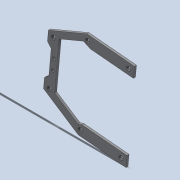
# Autodesk Inventor part: MuzzleHeadMount
Saved by Autodesk Inventor 2020 (Build 240168000, 168)
## iProperties
Created: 2021-07-18
Part Number: MuzzleHeadMount
Material: Generic
Document SubType Name: Sheet Metal
Designer: valer
Density: 1 g/cm^3
Sheet Metal Rule: Default
Appearance: Default
Author: valer
Autodesk Inventor part; units mm, degrees
ref_plane "YZ Plane" through (0, 0, 0) normal (1, 0, 0) x (0, 1, 0)
ref_plane "XZ Plane" through (0, 0, 0) normal (0, 1, 0) x (-1, 0, 0)
ref_plane "XY Plane" through (0, 0, 0) normal (0, 0, 1) x (1, 0, 0)
sketch "BottomBridge" plane through (0, 0, 0) normal (0, 0, -1) x (-1, 0, 0)
  ellipse E0 centre (-114.8689, -45.0046) end of major axis (-115.1437, -42.0173) minor radius 2.9795 (-113.78, -42.2136) -> (-113.289, -47.5501) ccw
  line L0 (-112.5709, -43.098) -> (-112.2615, -46.4599)
  line L1 (-57.1437, 12.2154) -> (-117.2531, 6.6843) construction
  line L2 (-117.2531, 6.6843) -> (-127.5262, -5.671)
  line L3 (-127.5262, -5.671) -> (-120.1358, -85.9876)
  line L4 (-120.1358, -85.9876) -> (-107.7805, -96.2608)
  line L5 (-118.7191, 22.617) -> (-138.253, 1.7684)
  line L6 (-138.253, 1.7684) -> (-129.3249, -95.2596)
  line L7 (-129.3249, -95.2596) -> (-106.3144, -112.1934)
  line L8 (-8.2453, 2.2991) -> (-1.4034, -72.0566) construction
  line L9 (-4.8244, -34.8788) -> (-133.7889, -46.7456) construction
  line L10 (-127.5262, -5.671) -> (-138.253, 1.7684) construction
  line L11 (-117.2531, 6.6843) -> (-118.7191, 22.617)
  line L12 (-118.7191, 22.617) -> (-117.2531, 6.6843)
  line L13 (-47.6711, -90.7297) -> (-107.7805, -96.2608)
  line L14 (-107.7805, -96.2608) -> (-106.3144, -112.1934)
  point P0 (0, 0)
  dimension "d29" = 9
  dimension "d30" = 10
  dimension "d31" = 50
  dimension "d32" = 135
  measures "d29" distance from line of L3 point (-114.869, -45.005)
  measures "d30" distance between parallel lines of L6 L3
  measures "d31" angle of L6 L10
  measures "d32" angle of L1 L2
sketch "Base" plane through (0, 0, 0) normal (0, 0, 1) x (1, 0, 0)
  circle A0 centre (0, 0) radius 3
  circle A1 centre (-6.2839, -68.2915) radius 2.875
  circle A2 centre (39.1052, -97.9753) radius 3
  circle A3 centre (99.0811, -103.4941) radius 3
  circle A4 centre (110.0198, 15.3837) radius 3
  circle A5 centre (50.0439, 20.9025) radius 3
  line L0 (-14.6913, -72.3521) -> (36.3914, -105.7594)
  line L1 (36.3914, -105.7594) -> (106.3144, -112.1934)
  line L2 (106.3144, -112.1934) -> (107.7805, -96.2608)
  line L3 (107.7805, -96.2608) -> (41.8191, -90.1913)
  line L4 (41.8191, -90.1913) -> (2.1235, -64.2309)
  line L5 (2.1235, -64.2309) -> (4.8244, -34.8788)
  line L6 (-178.2222, -18.0356) -> (255.5293, -57.9477) construction
  line L7 (-6.2839, -68.2915) -> (-3.142, -34.1457) construction
  line L8 (-6.2839, -68.2915) -> (39.1052, -97.9753) construction
  line L9 (39.1052, -97.9753) -> (99.0811, -103.4941) construction
  line L10 (-14.6913, -72.3521) -> (-11.1083, -33.4127)
  line L11 (4.8244, -34.8788) -> (-11.1083, -33.4127)
  line L12 (-7.5253, 5.5266) -> (48.7961, 29.0511)
  line L13 (48.7961, 29.0511) -> (118.7191, 22.617)
  line L14 (118.7191, 22.617) -> (117.2531, 6.6843)
  line L15 (117.2531, 6.6843) -> (51.2917, 12.7538)
  line L16 (51.2917, 12.7538) -> (7.5253, -5.5266)
  line L17 (7.5253, -5.5266) -> (4.8244, -34.8788)
  line L18 (-7.5253, 5.5266) -> (-11.1083, -33.4127)
  point P0 (0, 0)
  dimension "d0" = 8
  dimension "d1" = 8
  dimension "d2" = 8
  dimension "d3" = 8
  dimension "d4" = 8
  dimension "d5" = 8
  dimension "d6" = 8
  measures "d0" distance between parallel lines of L1 L9
  measures "d1" distance between parallel lines of L3 L9
  measures "d2" distance from line of L2 L9.end
  measures "d3" distance between parallel lines of L0 L8
  measures "d4" distance between parallel lines of L4 L8
  measures "d5" distance between parallel lines of L10 L7
  measures "d6" distance between parallel lines of L5 L7
extrude "Plate1" add sketch "Base" along normal blind 3.048
sketch "TopCut" plane through (0, 0, 3.048) normal (0, 0, 1) x (1, 0, 0)
  line L0 (-13.3312, -57.5708) -> (-6.8067, -52.1458)
  line L1 (-14.6913, -72.3521) -> (-7.5253, 5.5266) projected
  line L2 (7.5253, -5.5266) -> (2.1235, -64.2309) projected
  line L3 (-11.1083, -33.4127) -> (4.8244, -34.8788)
  line L4 (2.1235, -64.2309) -> (7.5253, -5.5266) projected
  line L5 (-6.8067, -52.1458) -> (-3.4604, -15.7791)
  line L6 (-3.4604, -15.7791) -> (-8.8854, -9.2546)
  point P0 (0, 0)
  point P1 (-5.1335, -33.9625)
  dimension "d8" = 45
  dimension "d9" = 45
  dimension "d10" = 6
  constraints: 8 end point, 3 midpoint, 3 point on line, 1 perpendicular
  measures "d8" angle of L1 L0
  measures "d9" angle of L1 L6
  measures "d10" distance between parallel lines of L1 L5
extrude "TopCutFeature" cut sketch "TopCut" against normal blind 3.048
sketch "SideCut" plane through (0, 0, 3.048) normal (0, 0, 1) x (1, 0, 0)
  ellipse E0 centre (35.8905, -88.6417) end of major axis (36.1653, -85.6543) minor radius 2.9795 (33.3641, -87.0543) -> (38.664, -87.542) ccw projected
  ellipse E1 centre (45.1798, 12.3117) end of major axis (44.9049, 9.3243) minor radius 2.9795 (42.6535, 13.8991) -> (47.9534, 13.4114) ccw projected
  line L0 (41.8191, -90.1913) -> (107.7805, -96.2608) projected
  line L1 (41.8191, -90.1913) -> (35.3649, -91.8772)
  line L2 (35.3649, -91.8772) -> (1.6108, -69.8026)
  line L3 (7.5253, -5.5266) -> (2.1235, -64.2309) projected
  line L4 (1.6108, -69.8026) -> (2.1235, -64.2309)
  line L5 (2.1235, -64.2309) -> (41.8191, -90.1913) construction
  line L6 (-178.2222, -18.0356) -> (255.5293, -57.9477)
  line L7 (41.8191, -90.1913) -> (2.1235, -64.2309)
  line L8 (51.2917, 12.7538) -> (45.2535, 15.5893)
  line L9 (45.2535, 15.5893) -> (8.0379, 0.045)
  line L10 (8.0379, 0.045) -> (7.5253, -5.5266)
  line L11 (7.5253, -5.5266) -> (51.2917, 12.7538)
  point P0 (0, 0)
  constraints: 18 end point, 3 symmetric about line, 1 collinear, 1 parallel, 7 other
extrude "SideCutFeature" cut sketch "SideCut" against normal blind 3.048 contours L2 L4 L7 E0 | E0 L1 L2 | E0 L7 L1 | L11 L10 L9 L8
sketch "MuzzleConnMountHoles" plane through (0, 0, 3.048) normal (0, 0, 1) x (1, 0, 0)
  line L0 (-3.4604, -15.7791) -> (-6.8067, -52.1458) projected
  line L1 (1.6108, -69.8026) -> (8.0379, 0.045) projected
  line L2 (-5.1335, -33.9625) -> (4.8244, -34.8788) construction
  line L3 (-6.8067, -52.1458) -> (-3.4604, -15.7791) projected
  circle A0 centre (-0.8876, -42.387) radius 2.5
  circle A1 centre (0.5785, -26.4543) radius 2.5
  line L4 (-0.8876, -42.387) -> (-0.1546, -34.4206) construction
  point P0 (0, 0)
  dimension "d15" = 5
  dimension "d24" = 8
  constraints: 4 end point, 3 midpoint, 2 centre point, 1 symmetric about line, 1 other
  measures "d15" diameter of A0
  measures "d24" distance of L4.start L4.end
hole "MuzzleConnMountHolesFeature" at (-0.8876, -42.387, 3.048) at (0.5785, -26.4543, 3.048) direction (0, 0, -1) diameter 4 depth 3.048 tip angle 118
sketch "SideCut2" plane through (0, 0, 0) normal (0, 0, -1) x (-1, 0, 0)
  ellipse E0 centre (-45.2535, 12.3052) end of major axis (-45.5283, 15.2925) minor radius 2.9795 (-43.3843, 9.9666) -> (-46.6644, 9.6648) ccw construction
  line L0 (-51.2917, 12.7538) -> (-117.2531, 6.6843) projected
  line L1 (-57.1437, 12.2154) -> (-45.301, 17.7766)
  line L2 (-45.301, 17.7766) -> (-8.2453, 2.2991)
  line L3 (-8.0379, 0.045) -> (-1.6108, -69.8026) projected
  line L4 (-8.2453, 2.2991) -> (-8.0379, 0.045)
  line L5 (-51.2917, 12.7538) -> (-45.2535, 15.5893) projected
  line L6 (-45.2535, 15.5893) -> (-8.0379, 0.045) projected
  line L7 (-1.6108, -69.8026) -> (-8.0379, 0.045) projected
  line L8 (-4.8244, -34.8788) -> (5.1335, -33.9625) construction
  line L9 (3.4604, -15.7791) -> (6.8067, -52.1458) projected
  line L10 (-47.6711, -90.7297) -> (-35.0124, -94.0364)
  line L11 (-35.0124, -94.0364) -> (-1.4034, -72.0566)
  line L12 (-1.4034, -72.0566) -> (-1.6108, -69.8026)
  line L13 (-1.6108, -69.8026) -> (-35.3649, -91.8772) projected
  line L14 (-35.3649, -91.8772) -> (-41.8191, -90.1913) projected
  line L15 (-107.7805, -96.2608) -> (-41.8191, -90.1913) projected
  point P0 (0, 0)
  dimension "d25" = 2
  dimension "d26" = 2
  constraints: 14 end point, 3 symmetric about line, 2 midpoint, 2 parallel, 1 collinear, 1 point on line, 1 other
  measures "d25" distance between parallel lines of L2 L6
  measures "d26" distance between parallel lines of L5 L1
extrude "SideCut2Feature" cut sketch "SideCut2" against normal blind 3.048
sheet face with bend "BottomBridgeFeature" sketch "BottomBridge" thickness 3.048 toward (0, 0, 1) bend radius 3.048 relief straight relief width 3.048 relief depth 1.524
bend "Bend1"
equation "\"d1\" = d0"
equation "\"d2\" = d0"
equation "\"d3\" = d0"
equation "\"d4\" = d0"
equation "\"d9\" = d8"
equation "\"d11\" = Thickness"
equation "\"d13\" = Thickness"
equation "\"d21\" = Thickness"
equation "\"d27\" = Thickness"
equation "\"d7\" = Thickness"
equation "\"d33\" = BendRadius"
equation "\"d34\" = BendReliefWidth"
equation "\"d36\" = MinimumRemnant"
equation "\"d35\" = BendReliefDepth"
equation "\"d37\" = TransitionRadius"
equation "\"BendRadius\" = Thickness"
equation "\"BendReliefWidth\" = Thickness"
equation "\"BendReliefDepth\" = 0.5 * Thickness"
equation "\"CornerReliefSize\" = 4 * Thickness"
equation "\"MinimumRemnant\" = 2 * Thickness"
equation "\"TransitionRadius\" = BendRadius"
equation "\"JacobiRadiusSize\" = BendRadius"
equation "\"GapSize\" = Thickness"
equation "\"Thickness\" = 3.048"
body "Solid1"
